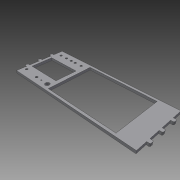
# Autodesk Inventor part: main_lcd_front_2
Saved by Autodesk Inventor 2014 (Build 180170000, 170)
## iProperties
Created: 2014-03-22
Part Number: main_lcd_front_2
Material: Plywood, Finish
Document SubType Name: Modeling
Designer: buben
Density: 0.552 g/cm^3
Appearance: Plywood - New
Author: buben
Autodesk Inventor part; units mm, degrees
ref_plane "YZ Plane" through (0, 0, 0) normal (1, 0, 0) x (0, 1, 0)
ref_plane "XZ Plane" through (0, 0, 0) normal (0, 1, 0) x (-1, 0, 0)
ref_plane "XY Plane" through (0, 0, 0) normal (0, 0, 1) x (1, 0, 0)
sketch "Sketch1" plane through (0, 0, 0) normal (0, 1, 0) x (-1, 0, 0)
  line L0 (0, 0) -> (-300, 0)
  line L1 (-300, 0) -> (-300, -120)
  line L2 (-300, -120) -> (0, -120)
  line L3 (0, -120) -> (0, 0)
  line L4 (-96.25, -114) -> (-258.25, -114)
  line L5 (-258.25, -114) -> (-258.25, -6)
  line L6 (-258.25, -6) -> (-96.25, -6)
  line L7 (-96.25, -6) -> (-96.25, -114)
  circle A0 centre (-10, -17.5) radius 3
  circle A1 centre (-49.075, -14.1) radius 3
  circle A2 centre (-64.25, -14.1) radius 1.5
  circle A3 centre (-83, -14.1) radius 5.5
  circle A4 centre (-64.25, -14.1) radius 5.85 construction
  line L8 (-46.075, -17.1) -> (-52.075, -17.1) construction
  line L9 (-52.075, -17.1) -> (-52.075, -11.1) construction
  line L10 (-52.075, -11.1) -> (-46.075, -11.1) construction
  line L11 (-46.075, -11.1) -> (-46.075, -17.1) construction
  line L12 (-76.25, -20.1) -> (-89.75, -20.1) construction
  line L13 (-89.75, -20.1) -> (-89.75, -8.1) construction
  line L14 (-89.75, -8.1) -> (-76.25, -8.1) construction
  line L15 (-76.25, -8.1) -> (-76.25, -20.1) construction
  line L16 (-7.75, -83.75) -> (-86.25, -83.75)
  line L17 (-86.25, -83.75) -> (-86.25, -32.25)
  line L18 (-86.25, -32.25) -> (-7.75, -32.25)
  line L19 (-7.75, -32.25) -> (-7.75, -83.75)
  line L20 (-8, -83.5) -> (-86, -83.5) construction
  line L21 (-86, -83.5) -> (-86, -32.5) construction
  line L22 (-86, -32.5) -> (-8, -32.5) construction
  line L23 (-8, -32.5) -> (-8, -83.5) construction
  line L24 (-0.5, -93) -> (-93.5, -93) construction
  line L25 (-93.5, -93) -> (-93.5, -6) construction
  line L26 (-93.5, -6) -> (-0.5, -6) construction
  line L27 (-0.5, -6) -> (-0.5, -93) construction
  point P0 (-49.075, -17.1)
  point P1 (-52.075, -14.1)
  point P2 (-83, -20.1)
  point P3 (-89.75, -14.1)
  point P4 (-47, -83.5)
  point P5 (-47, -83.75)
  point P6 (-86, -58)
  point P7 (-86.25, -58)
  dimension "d0" = 300
  dimension "d1" = 6
  dimension "d4" = 3
  dimension "d5" = 11
  dimension "d6" = 6
  dimension "d7" = 18.75
  dimension "d8" = 15.175
  dimension "d9" = 11.7
  dimension "d10" = 6
  dimension "d11" = 13.5
  dimension "d12" = 12
  dimension "d15" = 162
  dimension "d16" = 108
  dimension "d18" = 6
  dimension "d19" = 6
  dimension "d20" = 78.5
  dimension "d21" = 51.5
  dimension "d22" = 78
  dimension "d23" = 51
  dimension "d24" = 18.4
  dimension "d25" = 7.5
  dimension "d27" = 87
  dimension "d28" = 9.5
  dimension "d29" = 10
  dimension "d30" = 0.5
  dimension "d33" = 6
  dimension "d34" = 15
  dimension "d35" = 9.5
  dimension "d36" = 10.5
  dimension "d37" = 93
  constraints: 56 end point, 14 parallel, 8 midpoint, 8 perpendicular, 7 horizontal, 5 centre point, 5 horizontal alignment, 3 vertical alignment, 1 coincident
  measures "d0" distance of L0.start L0.end
  measures "d1" diameter of A0
  measures "d4" diameter of A2
  measures "d5" diameter of A3
  measures "d6" diameter of A1
  measures "d7" distance of A3.centre A2.centre
  measures "d8" distance of A2.centre A1.centre
  measures "d9" diameter of A4
  measures "d10" distance of L9.end L10.end
  measures "d11" distance of L13.end L14.end
  measures "d12" distance of L12.end L13.end
  measures "d15" distance of L5.end L6.end
  measures "d16" distance of L6.end L4.start
  measures "d18" distance between parallel lines of L6 L0
  measures "d19" distance between parallel lines of L2 L4
  measures "d20" distance of L17.end L18.end
  measures "d21" distance of L18.end L16.start
  measures "d22" distance of L21.end L22.end
  measures "d23" distance of L22.end L20.start
  measures "d24" vertical distance of L21.end A3.centre
  measures "d25" distance between parallel lines of L23 L27
  measures "d27" distance of L26.end L24.start
  measures "d28" distance between parallel lines of L24 L20
  measures "d29" distance between parallel lines of L17 L7
  measures "d30" distance between parallel lines of L3 L27
  measures "d33" distance between parallel lines of L0 L26
  measures "d34" distance from line of L22 A0.centre
  measures "d35" distance from line of A0.centre L27
  measures "d36" distance from line of L25 A3.centre
  measures "d37" distance of L24.start L24.end
extrude "Extrusion1" add sketch "Sketch1" along normal blind 6.5
sketch "Sketch2" plane through (0, 6.5, 0) normal (0, 1, 0) x (1, 0, 0)
  line L0 (7.75, 83.75) -> (86.25, 83.75) projected
  circle A0 centre (14.518, 104.846) radius 3
  circle A1 centre (32.775, 104.846) radius 3
  circle A2 centre (60.989, 104.846) radius 3
  circle A3 centre (78.996, 104.846) radius 3
  circle A4 centre (48.582, 104.846) radius 3
  circle A5 centre (80.796, 97.346) radius 1.5
  line L1 (9, 109.85) -> (85, 109.85) construction
  line L2 (85, 109.85) -> (85, 93.75) construction
  line L3 (85, 93.75) -> (9, 93.75) construction
  line L4 (9, 93.75) -> (9, 109.85) construction
  point P0 (47, 83.75)
  point P1 (47, 93.75)
  dimension "d38" = 6
  dimension "d39" = 18.257
  dimension "d40" = 15.807
  dimension "d41" = 12.407
  dimension "d42" = 18.007
  dimension "d43" = 3
  dimension "d44" = 1.8
  dimension "d45" = 7.5
  dimension "d46" = 76
  dimension "d47" = 16.1
  dimension "d48" = 5.004
  dimension "d49" = 5.518
  dimension "d50" = 10
  constraints: 8 end point, 6 centre point, 4 equal radius, 4 horizontal alignment, 2 midpoint, 2 parallel, 1 horizontal, 1 perpendicular, 1 vertical alignment
  measures "d38" diameter of A0
  measures "d39" distance of A1.centre A0.centre
  measures "d40" distance of A4.centre A1.centre
  measures "d41" distance of A2.centre A4.centre
  measures "d42" distance of A3.centre A2.centre
  measures "d43" diameter of A5
  measures "d44" horizontal distance of A5.centre A3.centre
  measures "d45" vertical distance of A5.centre A3.centre
  measures "d46" distance of L2.end L3.end
  measures "d47" distance of L3.end L1.start
  measures "d48" distance from line of A0.centre L1
  measures "d49" distance from line of L4 A0.centre
  measures "d50" distance between parallel lines of L0 L3
extrude "Extrusion2" cut sketch "Sketch2" against normal through all
sketch "Sketch3" plane through (0, 6.5, 0) normal (0, 1, 0) x (1, 0, 0)
  line L0 (0, 0) -> (300, 0) projected
  line L1 (300, 120) -> (0, 120) projected
  line L2 (0, 120) -> (0, 0) projected
  line L3 (0, 96) -> (-4.5, 96)
  line L4 (-6.5, 94) -> (-6.5, 90)
  line L5 (-4.5, 88) -> (0, 88)
  line L6 (0, 88) -> (0, 96)
  line L7 (0, 64) -> (-4.5, 64)
  line L8 (-6.5, 62) -> (-6.5, 58)
  line L9 (-4.5, 56) -> (0, 56)
  line L10 (0, 56) -> (0, 64)
  line L11 (0, 32) -> (-4.5, 32)
  line L12 (-6.5, 30) -> (-6.5, 26)
  line L13 (-4.5, 24) -> (0, 24)
  line L14 (0, 24) -> (0, 32)
  line L15 (150, 120) -> (150, 0) construction
  arc A0 (-4.5, 96) -> (-6.5, 94) centre (-4.5, 94) ccw
  arc A1 (-6.5, 90) -> (-4.5, 88) centre (-4.5, 90) ccw
  arc A2 (-4.5, 64) -> (-6.5, 62) centre (-4.5, 62) ccw
  arc A3 (-6.5, 58) -> (-4.5, 56) centre (-4.5, 58) ccw
  arc A4 (-4.5, 32) -> (-6.5, 30) centre (-4.5, 30) ccw
  arc A5 (-6.5, 26) -> (-4.5, 24) centre (-4.5, 26) ccw
  line L16 (-2.25, 96) -> (-2.25, 120) construction
  line L17 (-2.25, 88) -> (-2.25, 64) construction
  line L18 (-2.25, 56) -> (-2.25, 32) construction
  line L19 (-2.25, 24) -> (-2.25, 0) construction
  line L20 (300, 96) -> (304.5, 96)
  line L21 (306.5, 94) -> (306.5, 90)
  line L22 (304.5, 88) -> (300, 88)
  line L23 (300, 88) -> (300, 96)
  line L24 (300, 64) -> (304.5, 64)
  line L25 (306.5, 62) -> (306.5, 58)
  line L26 (304.5, 56) -> (300, 56)
  line L27 (300, 56) -> (300, 64)
  line L28 (300, 32) -> (304.5, 32)
  line L29 (306.5, 30) -> (306.5, 26)
  line L30 (304.5, 24) -> (300, 24)
  line L31 (300, 24) -> (300, 32)
  arc A6 (306.5, 94) -> (304.5, 96) centre (304.5, 94) ccw
  arc A7 (304.5, 88) -> (306.5, 90) centre (304.5, 90) ccw
  arc A8 (306.5, 62) -> (304.5, 64) centre (304.5, 62) ccw
  arc A9 (304.5, 56) -> (306.5, 58) centre (304.5, 58) ccw
  arc A10 (306.5, 30) -> (304.5, 32) centre (304.5, 30) ccw
  arc A11 (304.5, 24) -> (306.5, 26) centre (304.5, 26) ccw
  point P0 (302.25, 96)
  point P1 (302.25, 88)
  point P2 (302.25, 64)
  point P3 (302.25, 56)
  point P4 (302.25, 32)
  point P5 (302.25, 24)
  dimension "d53" = 2
  dimension "d54" = 8
  dimension "d55" = 8
  dimension "d56" = 8
  dimension "d57" = 6.5
  constraints: 58 end point, 30 symmetric about line, 24 point on circle, 12 centre point, 12 tangent, 8 midpoint, 7 parallel, 6 collinear, 5 equal radius, 3 horizontal, 3 perpendicular, 3 point on line, 2 horizontal alignment, 6 other
  measures "d53" radius of A0
  measures "d54" distance between parallel lines of L5 L3
  measures "d55" distance between parallel lines of L9 L7
  measures "d56" distance between parallel lines of L13 L11
  measures "d57" distance between parallel lines of L2 L4
extrude "Extrusion3" add sketch "Sketch3" against normal blind 6.5
sketch "Sketch4" plane through (0, 6.5, 0) normal (0, 1, 0) x (1, 0, 0)
  circle A0 centre (80.796, 97.346) radius 1.5 projected
extrude "Extrusion4" add sketch "Sketch4" against normal blind 6.5
body "Solid1"
